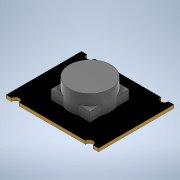
# Autodesk Inventor part: Camera
Saved by Autodesk Inventor 2022 (Build 260153000, 153)
## iProperties
Created: 2021-11-09
Part Number: Camera
Material: Generic
Document SubType Name: Modeling
Designer: Juan
Density: 1 g/cm^3
Appearance: Default
Author: Juan
Autodesk Inventor part; units mm, degrees
ref_plane "YZ Plane" through (0, 0, 0) normal (1, 0, 0) x (0, 1, 0)
ref_plane "XZ Plane" through (0, 0, 0) normal (0, 1, 0) x (-1, 0, 0)
ref_plane "XY Plane" through (0, 0, 0) normal (0, 0, 1) x (1, 0, 0)
sketch "Sketch1" plane through (0, 0, 0) normal (0, 1, 0) x (-1, 0, 0)
  line L0 (-15, 12.25) -> (15, 12.25)
  line L1 (15, 12.25) -> (15, -12.25)
  line L2 (15, -12.25) -> (-15, -12.25)
  line L3 (-15, -12.25) -> (-15, 12.25)
  line L4 (-15, 12.25) -> (15, -12.25) construction
  line L5 (15, 12.25) -> (-15, -12.25) construction
  line L6 (-12, 12.25) -> (12, 12.25)
  line L7 (12, 12.25) -> (12, -12.25)
  line L8 (12, -12.25) -> (-12, -12.25)
  line L9 (-12, -12.25) -> (-12, 12.25)
  line L10 (-12, 12.25) -> (12, -12.25) construction
  line L11 (12, 12.25) -> (-12, -12.25) construction
  circle A0 centre (12, -12.25) radius 1.25
  circle A1 centre (-12, -12.25) radius 1.25
  circle A2 centre (-12, 12.25) radius 1.25
  circle A3 centre (12, 12.25) radius 1.25
  point P0 (0, 0)
  point P1 (13.25, 12.25)
  point P2 (10.75, 12.25)
  point P3 (-10.75, 12.25)
  point P4 (-13.25, 12.25)
  point P5 (-13.25, -12.25)
  point P6 (-10.75, -12.25)
  point P7 (10.75, -12.25)
  point P8 (13.25, -12.25)
  dimension "d0" = 30
  dimension "d1" = 24.5
  dimension "d2" = 24
  dimension "d3" = 2.5
  constraints: 24 end point, 4 centre point, 4 coincident, 4 midpoint, 4 parallel, 3 equal radius, 2 horizontal, 2 perpendicular, 1 point on line
  measures "d0" distance of L1.end L2.end
  measures "d1" distance of L0.end L1.end
  measures "d2" distance of L7.end L8.end
  measures "d3" diameter of A0
extrude "Extrusion1" add sketch "Sketch1" along normal blind 1 contours L0 A3 L7 A0 L2 A1 L9 A2 | A2 L9 A1 L2 L3 L0 | L0 L1 L2 A0 L7 A3
sketch "Sketch2" plane through (0, 1, 0) normal (0, 1, 0) x (1, 0, 0)
  line L0 (-6.3, 6.3) -> (6.3, 6.3)
  line L1 (6.3, 6.3) -> (6.3, -6.3)
  line L2 (6.3, -6.3) -> (-6.3, -6.3)
  line L3 (-6.3, -6.3) -> (-6.3, 6.3)
  line L4 (-6.3, 6.3) -> (6.3, -6.3) construction
  line L5 (6.3, 6.3) -> (-6.3, -6.3) construction
  point P0 (0, 0)
  dimension "d6" = 12.6
  dimension "d7" = 12.6
  constraints: 12 end point, 2 midpoint, 2 parallel, 1 horizontal, 1 perpendicular
  measures "d6" distance of L1.end L2.end
  measures "d7" distance of L0.end L1.end
extrude "Extrusion2" add sketch "Sketch2" along normal blind 3
sketch "Sketch3" plane through (0, 4, 0) normal (0, 1, 0) x (1, 0, 0)
  circle A0 centre (0, 0) radius 6.75
  dimension "d10" = 13.5
  constraints: 1 centre point, 1 coincident
  measures "d10" diameter of A0
extrude "Extrusion3" add sketch "Sketch3" along normal blind 3.5 and the other way blind 3
body "Solid1"
